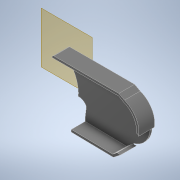
# Autodesk Inventor part: Pieza4_Carcasa
Saved by Autodesk Inventor 2022 (Build 260153000, 153)
## iProperties
Created: 2022-11-06
Part Number: Pieza4_Carcasa
Material: Resina acetálica, negra
Document SubType Name: Modeling
Designer: Mauricio Guerrero
Density: 1.425 g/cm^3
Appearance: Suave - Negro
Author: Mauricio Guerrero
## iProperties of the stored document Pieza4_Carcasa_3DPrint.ipt
Created: 2022-11-06
Part Number: Pieza4_Carcasa_3DPrint
Material: Genérico
Document SubType Name: Modeling
Designer: Mauricio Guerrero
Density: 1 g/cm^3
Appearance: Valor por defecto
Author: Mauricio Guerrero
Autodesk Inventor part; units mm, degrees
ref_plane "YZ Plane" through (0, 0, 0) normal (1, 0, 0) x (0, 1, 0)
ref_plane "XZ Plane" through (0, 0, 0) normal (0, 1, 0) x (-1, 0, 0)
ref_plane "XY Plane" through (0, 0, 0) normal (0, 0, 1) x (1, 0, 0)
ref_plane "Plano de trabajo2" through (0, 0, 6) normal (0, 0, 1) x (1, 0, 0)
sketch "Boceto2" plane through (0, 0, 6) normal (0, 0, 1) x (1, 0, 0)
  line L0 (3.4877, 0.0061) -> (2.356, 0.0061)
  line L1 (-0.3158, 0.0061) -> (3.4877, 0.0061)
  line L2 (2.3154, 0.578) -> (3.4274, 0.0367)
  line L3 (3.4877, 0.0061) -> (2.3154, 0.578)
  line L4 (0.839, 0.7797) -> (1.4401, 0.7797)
  line L5 (0.839, 0.7797) -> (1.4401, 0.7797)
  arc A0 (1.265, 1.6527) -> (0.7783, 1.0384) centre (1.265, 1.1527) ccw
  line L6 (1.265, 1.6527) -> (29.2586, 1.6527)
  line L7 (29.2586, 1.6527) -> (31.3921, 0.3915)
  arc A1 (29.9614, -18.679) -> (36.7928, -8.9256) centre (27.2383, -9.5026) ccw
  line L8 (29.9614, -18.679) -> (26.6305, -21.3323)
  line L9 (26.6305, -21.3323) -> (8.816, -21.0119)
  line L10 (8.816, -21.0119) -> (8.8579, -18.68)
  arc A2 (9.226, -15.1503) -> (5.8136, -13.2096) centre (6.1366, -16.6121) ccw
  arc A3 (8.8579, -18.68) -> (9.226, -15.1503) centre (-12.417, -14.6773) ccw
  line L11 (0.839, 0.7797) -> (0.7783, 1.0384)
  line L12 (0.839, 0.7797) -> (0.7783, 1.0384)
  arc A4 (2.3154, 0.578) -> (1.4401, 0.7797) centre (1.4401, -1.2203) ccw
  arc A5 (2.3154, 0.578) -> (1.4401, 0.7797) centre (1.4401, -1.2203) ccw
  arc A6 (1.265, 1.6527) -> (0.7783, 1.0384) centre (1.265, 1.1527) ccw
  arc A7 (36.7928, -8.9256) -> (31.3921, 0.3915) centre (28.668, -7.4114) ccw
  arc A8 (9.226, -15.1503) -> (5.8136, -13.2096) centre (6.1366, -16.6121) ccw
  arc A9 (5.8136, -13.2096) -> (1.6377, -1.6896) centre (-9.1156, -12.1045) ccw
  arc A10 (2.356, 0.0061) -> (1.6377, -1.6896) centre (2.356, -0.9939) ccw
  point P0 (0, 0)
  point P1 (0, 0)
  dimension "d15" = 1
  constraints: 26 end point, 23 point on circle, 11 centre point, 3 collinear, 3 tangent, 1 concentric, 1 horizontal, 1 perpendicular, 1 point on line
  measures "d15" radius of A10
extrude "Extrusión2" add sketch "Boceto2" along normal blind 0.8
ref_plane "Plano de trabajo1" through (0, 0, 6) normal (0, 0, 1) x (1, 0, 0)
sketch "Boceto3" plane through (0, 0, 6) normal (0, 0, 1) x (1, 0, 0)
  line L0 (1.265, 1.6527) -> (29.2586, 1.6527)
  line L1 (1.265, 1.6527) -> (29.2586, 1.6527)
  line L2 (8.816, -21.0119) -> (26.6305, -21.3323)
  line L3 (31.3921, 0.3915) -> (29.2586, 1.6527)
  line L4 (29.2586, 1.6527) -> (31.3921, 0.3915)
  arc A0 (36.8741, -8.3478) -> (31.361, 0.4098) centre (28.554, -7.4714) ccw
  line L5 (26.6305, -21.3323) -> (28.554, -19.8001)
  arc A1 (1.265, 1.6527) -> (0.7783, 1.0384) centre (1.265, 1.1527) ccw
  arc A2 (1.265, 1.6527) -> (0.7783, 1.0384) centre (1.265, 1.1527) ccw
  line L6 (8.816, -22.0121) -> (26.9722, -22.3386)
  line L7 (26.9722, -22.3386) -> (30.1015, -19.8459)
  arc A3 (37.7776, -9.0994) -> (31.6965, 1.3519) centre (28.554, -7.4714) ccw
  line L8 (1.265, 2.6527) -> (29.2586, 2.6527)
  line L9 (8.816, -22.0121) -> (8.816, -21.0119)
  arc A4 (1.265, 2.6527) -> (0.4911, 1.8106) centre (1.4694, 1.6882) ccw
  line L10 (0.4911, 1.8106) -> (0.6535, 1.5698)
  line L11 (0.6535, 1.5698) -> (1.265, 1.6527)
  line L12 (29.2586, 2.6527) -> (31.6965, 1.3519)
  arc A5 (28.554, -19.8001) -> (30.1015, -19.8459) centre (29.4255, -16.5211) ccw
  arc A6 (37.7776, -9.0994) -> (36.8741, -8.3478) centre (36.907, -9.227) ccw
  point P0 (0, 0)
  point P1 (0, 0)
  point P2 (-0.3158, 0.0061)
  point P3 (-7.6246, -8.019)
  point P4 (-11.4954, -7.0855)
  point P5 (1.132, 1.6347)
  point P6 (31.361, 0.4098)
  dimension "d10" = 1
  dimension "d11" = 1
  dimension "d12" = 1
  constraints: 26 end point, 14 point on circle, 7 centre point, 2 equal length, 1 horizontal, 1 point on line, 1 vertical
  measures "d10" distance between parallel lines of L2 L6
  measures "d11" radial gap between concentric circles of A0 A3
  measures "d12" distance between parallel lines of L0 L8
extrude "Extrusión3" add sketch "Boceto3" along normal blind 6.8
